Autodesk Inventor part; units mm, degrees
(part 2 of 3)
  line L643 (23.995, -22.9988) -> (23.995, -46.9725)
  line L644 (23.995, -46.9725) -> (32, -46.9725)
  line L645 (32, -46.9725) -> (40.005, -46.9725)
  line L646 (40.005, -46.9725) -> (41.9959, -46.9725)
  line L647 (41.9959, -46.9725) -> (48.01, -40.9997)
  line L648 (48.01, -40.9997) -> (48.01, -22.9988)
  line L649 (32, -47.4798) -> (32.0841, -48.285)
  line L650 (32.0841, -48.285) -> (32.3378, -49.0047)
  line L651 (32.3378, -49.0047) -> (32.6769, -49.7258)
  line L652 (32.6769, -49.7258) -> (33.1857, -50.3187)
  line L653 (33.1857, -50.3187) -> (33.7786, -50.826)
  line L654 (33.7786, -50.826) -> (34.4983, -51.1652)
  line L655 (34.4983, -51.1652) -> (35.218, -51.4189)
  line L656 (35.218, -51.4189) -> (36.0232, -51.5044)
  line L657 (36.0232, -51.5044) -> (36.7856, -51.4189)
  line L658 (36.7856, -51.4189) -> (37.548, -51.1652)
  line L659 (37.548, -51.1652) -> (38.225, -50.826)
  line L660 (38.225, -50.826) -> (38.8606, -50.3187)
  line L661 (38.8606, -50.3187) -> (39.3266, -49.7258)
  line L662 (39.3266, -49.7258) -> (39.7085, -49.0047)
  line L663 (39.7085, -49.0047) -> (39.9195, -48.285)
  line L664 (39.9195, -48.285) -> (40.005, -47.4798)
  line L665 (40.005, -22.4915) -> (39.9195, -21.729)
  line L666 (39.9195, -21.729) -> (39.7085, -20.9666)
  line L667 (39.7085, -20.9666) -> (39.3266, -20.2455)
  line L668 (39.3266, -20.2455) -> (38.8606, -19.6526)
  line L669 (38.8606, -19.6526) -> (38.225, -19.1453)
  line L670 (38.225, -19.1453) -> (37.548, -18.8061)
  line L671 (37.548, -18.8061) -> (36.7856, -18.5524)
  line L672 (36.7856, -18.5524) -> (36.0232, -18.5096)
  line L673 (36.0232, -18.5096) -> (35.218, -18.5524)
  line L674 (35.218, -18.5524) -> (34.4983, -18.8061)
  line L675 (34.4983, -18.8061) -> (33.7786, -19.1453)
  line L676 (33.7786, -19.1453) -> (33.1857, -19.6526)
  line L677 (33.1857, -19.6526) -> (32.6769, -20.2455)
  line L678 (32.6769, -20.2455) -> (32.3378, -20.9666)
  line L679 (32.3378, -20.9666) -> (32.0841, -21.729)
  line L680 (32.0841, -21.729) -> (32, -22.4915)
  line L681 (40.005, -47.4798) -> (40.005, -46.9725)
  line L682 (32, -47.4798) -> (32, -46.9725)
  line L683 (40.005, -22.4915) -> (40.005, -22.9988)
  line L684 (32, -22.4915) -> (32, -22.9988)
  line L685 (-48.9834, -46.9725) -> (-40.9784, -46.9725)
  line L686 (-40.9784, -46.9725) -> (-32.9734, -46.9725)
  line L687 (-32.9734, -46.9725) -> (-25.0111, -46.9725)
  line L688 (-25.0111, -46.9725) -> (-25.0111, -22.9988)
  line L689 (-25.0111, -22.9988) -> (-32.9734, -22.9988)
  line L690 (-32.9734, -22.9988) -> (-40.9784, -22.9988)
  line L691 (-40.9784, -22.9988) -> (-43.012, -22.9988)
  line L692 (-43.012, -22.9988) -> (-48.9834, -28.9716)
  line L693 (-48.9834, -28.9716) -> (-48.9834, -46.9725)
  line L694 (-32.9734, -22.4915) -> (-33.0575, -21.729)
  line L695 (-33.0575, -21.729) -> (-33.3126, -20.9666)
  line L696 (-33.3126, -20.9666) -> (-33.6503, -20.2455)
  line L697 (-33.6503, -20.2455) -> (-34.1591, -19.6526)
  line L698 (-34.1591, -19.6526) -> (-34.752, -19.1453)
  line L699 (-34.752, -19.1453) -> (-35.4717, -18.8061)
  line L700 (-35.4717, -18.8061) -> (-36.1927, -18.5524)
  line L701 (-36.1927, -18.5524) -> (-36.9965, -18.5096)
  line L702 (-36.9965, -18.5096) -> (-37.759, -18.5524)
  line L703 (-37.759, -18.5524) -> (-38.5214, -18.8061)
  line L704 (-38.5214, -18.8061) -> (-39.1998, -19.1453)
  line L705 (-39.1998, -19.1453) -> (-39.8354, -19.6526)
  line L706 (-39.8354, -19.6526) -> (-40.3, -20.2455)
  line L707 (-40.3, -20.2455) -> (-40.6819, -20.9666)
  line L708 (-40.6819, -20.9666) -> (-40.8943, -21.729)
  line L709 (-40.8943, -21.729) -> (-40.9784, -22.4915)
  line L710 (-40.9784, -47.4798) -> (-40.8943, -48.285)
  line L711 (-40.8943, -48.285) -> (-40.6819, -49.0047)
  line L712 (-40.6819, -49.0047) -> (-40.3, -49.7258)
  line L713 (-40.3, -49.7258) -> (-39.8354, -50.3187)
  line L714 (-39.8354, -50.3187) -> (-39.1998, -50.826)
  line L715 (-39.1998, -50.826) -> (-38.5214, -51.1652)
  line L716 (-38.5214, -51.1652) -> (-37.759, -51.4189)
  line L717 (-37.759, -51.4189) -> (-36.9965, -51.5044)
  line L718 (-36.9965, -51.5044) -> (-36.1927, -51.4189)
  line L719 (-36.1927, -51.4189) -> (-35.4717, -51.1652)
  line L720 (-35.4717, -51.1652) -> (-34.752, -50.826)
  line L721 (-34.752, -50.826) -> (-34.1591, -50.3187)
  line L722 (-34.1591, -50.3187) -> (-33.6503, -49.7258)
  line L723 (-33.6503, -49.7258) -> (-33.3126, -49.0047)
  line L724 (-33.3126, -49.0047) -> (-33.0575, -48.285)
  line L725 (-33.0575, -48.285) -> (-32.9734, -47.4798)
  line L726 (-40.9784, -22.4915) -> (-40.9784, -22.9988)
  line L727 (-32.9734, -22.4915) -> (-32.9734, -22.9988)
  line L728 (-40.9784, -47.4798) -> (-40.9784, -46.9725)
  line L729 (-32.9734, -47.4798) -> (-32.9734, -46.9725)
  line L730 (-22.9775, -13.469) -> (-22.9775, 13.5103)
  line L731 (-22.9775, 13.5103) -> (-4.9766, 13.5103)
  line L732 (-4.9766, 13.5103) -> (-4.9766, -13.469)
  line L733 (-4.9766, -13.469) -> (-22.9775, -13.469)
  line L734 (-22.0027, -6.4801) -> (-18.9957, -6.4801)
  line L735 (-20.4778, -4.998) -> (-20.4778, -8.005)
  line L736 (-20.4778, 8.005) -> (-20.4778, 4.9979)
  line L737 (-2.9857, -15.333) -> (3.1553, -15.333)
  line L738 (3.1553, -15.333) -> (3.1553, -17.4935)
  line L739 (3.1553, -17.4935) -> (-2.9857, -17.4935)
  line L740 (-2.9857, -17.4935) -> (-2.9857, -15.333)
  line L741 (-0.7411, -15.5453) -> (-0.7411, -17.2812)
  line L742 (0.7838, -16.3919) -> (-0.7411, -15.5453)
  line L743 (-0.7411, -17.2812) -> (0.7838, -16.3919)
  line L744 (0.7838, -15.5453) -> (0.7838, -16.3919)
  line L745 (0.7838, -16.3919) -> (0.7838, -17.2812)
  line L746 (-4.1714, 19.4403) -> (-4.1714, 19.1866)
  line L747 (-4.1714, 19.1866) -> (-4.1714, 16.2637)
  line L748 (-4.1714, 16.2637) -> (0.2751, 16.2637)
  line L749 (0.2751, 16.2637) -> (0.2751, 19.4403)
  line L750 (0.2751, 19.4403) -> (-3.7909, 19.4403)
  line L751 (-3.7909, 19.4403) -> (-3.875, 19.4403)
  line L752 (-3.875, 19.4403) -> (-4.1714, 19.4403)
  line L753 (-3.875, 19.4403) -> (-3.875, 19.1866)
  line L754 (-3.875, 19.1866) -> (-4.1714, 19.1866)
  line L755 (-3.7909, 19.4403) -> (-3.7909, 19.1439)
  line L756 (-3.7909, 19.1439) -> (-4.0873, 19.1439)
  line L757 (64.104, 31.9772) -> (64.104, 33.6717)
  line L758 (50.6351, 31.9772) -> (50.6351, 33.6717)
  line L759 (64.104, 14.1032) -> (63.1307, 14.1032)
  line L760 (64.104, 14.1032) -> (64.104, 15.0779)
  line L761 (50.6351, 14.1032) -> (51.6099, 14.1032)
  line L762 (50.6351, 14.1032) -> (50.6351, 15.0779)
  line L763 (50.6351, 39.8981) -> (51.6099, 39.8981)
  line L764 (50.6351, 39.8981) -> (50.6351, 38.882)
  line L765 (64.104, 39.8981) -> (63.0038, 39.8981)
  line L766 (64.104, 39.8981) -> (64.104, 38.882)
  line L767 (-5.9927, -49.9795) -> (5.9941, -49.9795)
  line L768 (5.9941, -49.9795) -> (5.9941, -48.9634)
  line L769 (5.9941, -48.9634) -> (5.9941, -38.9675)
  line L770 (5.9941, -38.9675) -> (5.9941, -29.9877)
  line L771 (5.9941, -29.9877) -> (-5.9927, -29.9877)
  line L772 (-5.9927, -29.9877) -> (-5.9927, -38.9675)
  line L773 (-5.9927, -38.9675) -> (-5.9927, -48.9634)
  line L774 (-5.9927, -48.9634) -> (-5.9927, -49.9795)
  line L775 (-8.9998, -38.9675) -> (-9.8477, -39.0516)
  line L776 (-9.8477, -39.0516) -> (-10.6942, -39.2639)
  line L777 (-10.6942, -39.2639) -> (-11.4994, -39.6444)
  line L778 (-11.4994, -39.6444) -> (-12.2191, -40.1532)
  line L779 (-12.2191, -40.1532) -> (-12.812, -40.746)
  line L780 (-12.812, -40.746) -> (-13.3207, -41.4658)
  line L781 (-13.3207, -41.4658) -> (-13.7013, -42.2709)
  line L782 (-13.7013, -42.2709) -> (-13.9136, -43.1175)
  line L783 (-13.9136, -43.1175) -> (-13.9977, -43.9654)
  line L784 (-13.9977, -43.9654) -> (-13.9136, -44.8547)
  line L785 (-13.9136, -44.8547) -> (-13.7013, -45.7013)
  line L786 (-13.7013, -45.7013) -> (-13.3207, -46.4637)
  line L787 (-13.3207, -46.4637) -> (-12.812, -47.1834)
  line L788 (-12.812, -47.1834) -> (-12.2191, -47.819)
  line L789 (-12.2191, -47.819) -> (-11.4994, -48.3278)
  line L790 (-11.4994, -48.3278) -> (-10.6942, -48.6669)
  line L791 (-10.6942, -48.6669) -> (-9.8477, -48.9206)
  line L792 (-9.8477, -48.9206) -> (-8.9998, -48.9634)
  line L793 (9.0011, -48.9634) -> (9.8904, -48.9206)
  line L794 (9.8904, -48.9206) -> (10.737, -48.6669)
  line L795 (10.737, -48.6669) -> (11.4994, -48.3278)
  line L796 (11.4994, -48.3278) -> (12.2191, -47.819)
  line L797 (12.2191, -47.819) -> (12.8547, -47.1834)
  line L798 (12.8547, -47.1834) -> (13.3635, -46.4637)
  line L799 (13.3635, -46.4637) -> (13.7027, -45.7013)
  line L800 (13.7027, -45.7013) -> (13.9563, -44.8547)
  line L801 (13.9563, -44.8547) -> (13.9991, -43.9654)
  line L802 (13.9991, -43.9654) -> (13.9563, -43.1175)
  line L803 (13.9563, -43.1175) -> (13.7027, -42.2709)
  line L804 (13.7027, -42.2709) -> (13.3635, -41.4658)
  line L805 (13.3635, -41.4658) -> (12.8547, -40.746)
  line L806 (12.8547, -40.746) -> (12.2191, -40.1532)
  line L807 (12.2191, -40.1532) -> (11.4994, -39.6444)
  line L808 (11.4994, -39.6444) -> (10.737, -39.2639)
  line L809 (10.737, -39.2639) -> (9.8904, -39.0516)
  line L810 (9.8904, -39.0516) -> (9.0011, -38.9675)
  line L811 (-8.9998, -38.9675) -> (-5.9927, -38.9675)
  line L812 (-8.9998, -48.9634) -> (-5.9927, -48.9634)
  line L813 (5.9941, -38.9675) -> (9.0011, -38.9675)
  line L814 (5.9941, -48.9634) -> (9.0011, -48.9634)
  line L815 (-7.4749, -49.9795) -> (-7.4749, -38.4587)
  line L816 (-7.4749, -38.4587) -> (7.5176, -38.4587)
  line L817 (7.5176, -38.4587) -> (7.5176, -49.9795)
  line L818 (7.5176, -49.9795) -> (-7.4749, -49.9795)
  line L819 (5.9941, 49.9781) -> (-5.9927, 49.9781)
  line L820 (-5.9927, 49.9781) -> (-5.9927, 49.0047)
  line L821 (-5.9927, 49.0047) -> (-5.9927, 39.0088)
  line L822 (-5.9927, 39.0088) -> (-5.9927, 29.9863)
  line L823 (-5.9927, 29.9863) -> (5.9941, 29.9863)
  line L824 (5.9941, 29.9863) -> (5.9941, 39.0088)
  line L825 (5.9941, 39.0088) -> (5.9941, 49.0047)
  line L826 (5.9941, 49.0047) -> (5.9941, 49.9781)
  line L827 (9.0011, 39.0088) -> (9.8904, 39.0929)
  line L828 (9.8904, 39.0929) -> (10.737, 39.3053)
  line L829 (10.737, 39.3053) -> (11.4994, 39.6858)
  line L830 (11.4994, 39.6858) -> (12.2191, 40.1518)
  line L831 (12.2191, 40.1518) -> (12.8547, 40.7874)
  line L832 (12.8547, 40.7874) -> (13.3635, 41.5071)
  line L833 (13.3635, 41.5071) -> (13.7027, 42.2696)
  line L834 (13.7027, 42.2696) -> (13.9563, 43.1175)
  line L835 (13.9563, 43.1175) -> (13.9991, 44.0068)
  line L836 (13.9991, 44.0068) -> (13.9563, 44.8533)
  line L837 (13.9563, 44.8533) -> (13.7027, 45.7013)
  line L838 (13.7027, 45.7013) -> (13.3635, 46.5051)
  line L839 (13.3635, 46.5051) -> (12.8547, 47.2261)
  line L840 (12.8547, 47.2261) -> (12.2191, 47.819)
  line L841 (12.2191, 47.819) -> (11.4994, 48.3264)
  line L842 (11.4994, 48.3264) -> (10.737, 48.7083)
  line L843 (10.737, 48.7083) -> (9.8904, 48.9192)
  line L844 (9.8904, 48.9192) -> (9.0011, 49.0047)
  line L845 (-8.9998, 49.0047) -> (-9.8477, 48.9192)
  line L846 (-9.8477, 48.9192) -> (-10.6942, 48.7083)
  line L847 (-10.6942, 48.7083) -> (-11.4994, 48.3264)
  line L848 (-11.4994, 48.3264) -> (-12.2191, 47.819)
  line L849 (-12.2191, 47.819) -> (-12.812, 47.2261)
  line L850 (-12.812, 47.2261) -> (-13.3207, 46.5051)
  line L851 (-13.3207, 46.5051) -> (-13.7013, 45.7013)
  line L852 (-13.7013, 45.7013) -> (-13.9136, 44.8533)
  line L853 (-13.9136, 44.8533) -> (-13.9977, 44.0068)
  line L854 (-13.9977, 44.0068) -> (-13.9136, 43.1175)
  line L855 (-13.9136, 43.1175) -> (-13.7013, 42.2696)
  line L856 (-13.7013, 42.2696) -> (-13.3207, 41.5071)
  line L857 (-13.3207, 41.5071) -> (-12.812, 40.7874)
  line L858 (-12.812, 40.7874) -> (-12.2191, 40.1518)
  line L859 (-12.2191, 40.1518) -> (-11.4994, 39.6858)
  line L860 (-11.4994, 39.6858) -> (-10.6942, 39.3053)
  line L861 (-10.6942, 39.3053) -> (-9.8477, 39.0929)
  line L862 (-9.8477, 39.0929) -> (-8.9998, 39.0088)
  line L863 (9.0011, 39.0088) -> (5.9941, 39.0088)
  line L864 (9.0011, 49.0047) -> (5.9941, 49.0047)
  line L865 (-5.9927, 39.0088) -> (-8.9998, 39.0088)
  line L866 (-5.9927, 49.0047) -> (-8.9998, 49.0047)
  line L867 (7.5176, 49.9781) -> (7.5176, 38.5001)
  line L868 (7.5176, 38.5001) -> (-7.4749, 38.5001)
  line L869 (-7.4749, 38.5001) -> (-7.4749, 49.9781)
  line L870 (-7.4749, 49.9781) -> (7.5176, 49.9781)
  line L871 (29.2894, -9.1066) -> (32.5928, -9.1066)
  line L872 (32.5928, -9.1066) -> (32.5928, -14.3169)
  line L873 (32.5928, -14.3169) -> (29.2894, -14.3169)
  line L874 (29.2894, -14.3169) -> (29.2894, -9.1066)
  line L875 (31.0679, -4.1941) -> (31.0679, 2.7947)
  line L876 (31.0679, 2.7947) -> (38.0568, 2.7947)
  line L877 (38.0568, 2.7947) -> (38.0568, -3.855)
  line L878 (37.7176, -4.1941) -> (31.0679, -4.1941)
  line L879 (37.7176, -4.1941) -> (38.0568, -3.855)
  line L880 (58.0472, -22.5328) -> (68.2554, -22.5328)
  line L881 (68.2554, -22.5328) -> (68.2554, -17.3239)
  line L882 (68.2554, -17.3239) -> (58.0472, -17.3239)
  line L883 (58.0472, -17.3653) -> (58.0472, -21.1775)
  line L884 (58.0472, -21.1775) -> (58.0472, -22.4487)
  line L885 (59.3184, -22.4487) -> (59.3184, -21.1775)
  line L886 (59.3184, -21.1775) -> (58.0472, -21.1775)
  line L887 (68.0018, -3.9818) -> (68.0018, -1.1016)
  line L888 (68.0018, -1.1016) -> (69.8644, -1.1016)
  line L889 (69.8644, -1.1016) -> (69.8644, -3.9818)
  line L890 (69.8644, -3.9818) -> (68.0018, -3.9818)
  line L891 (49.2798, 0.1696) -> (49.1957, 0.6356)
  line L892 (49.1957, 0.6356) -> (49.0261, 1.1002)
  line L893 (49.0261, 1.1002) -> (48.7724, 1.5249)
  line L894 (48.7724, 1.5249) -> (48.3905, 1.8213)
  line L895 (48.3905, 2.4555) -> (49.408, 2.4555)
  line L896 (48.3905, -8.3869) -> (48.7724, -8.0477)
  line L897 (48.7724, -8.0477) -> (49.0261, -7.6672)
  line L898 (49.0261, -7.6672) -> (49.1957, -7.2012)
  line L899 (49.1957, -7.2012) -> (49.2798, -6.6924)
  line L900 (48.3905, -8.9798) -> (49.408, -8.9798)
  line L901 (45.9763, -6.6924) -> (45.9763, 0.1696)
  line L902 (45.2139, -6.6924) -> (45.2139, 0.1696)
  line L903 (48.5173, 0.1696) -> (48.5173, -6.6924)
  line L904 (44.8333, -8.7261) -> (44.8333, 2.2019)
  line L905 (44.8333, -8.7261) -> (44.8747, -8.8529)
  line L906 (44.8747, -8.8529) -> (44.9602, -8.937)
  line L907 (44.9602, -8.937) -> (45.087, -8.9798)
  line L908 (45.087, -8.9798) -> (46.1032, -8.9798)
  line L909 (45.9763, -6.6924) -> (46.0191, -6.9889)
  line L910 (46.0191, -6.9889) -> (46.1032, -7.2425)
  line L911 (48.3905, -7.2425) -> (48.476, -6.9889)
  line L912 (48.476, -6.9889) -> (48.5173, -6.6924)
  line L913 (45.2139, -6.6924) -> (45.2566, -7.2012)
  line L914 (45.2566, -7.2012) -> (45.4262, -7.6672)
  line L915 (45.4262, -7.6672) -> (45.7226, -8.0477)
  line L916 (45.7226, -8.0477) -> (46.1032, -8.3869)
  line L917 (46.1032, 1.8213) -> (45.7226, 1.5249)
  line L918 (45.7226, 1.5249) -> (45.4262, 1.1002)
  line L919 (45.4262, 1.1002) -> (45.2566, 0.6356)
  line L920 (45.2566, 0.6356) -> (45.2139, 0.1696)
  line L921 (46.1032, 0.7197) -> (46.0191, 0.466)
  line L922 (46.0191, 0.466) -> (45.9763, 0.1696)
  line L923 (48.5173, 0.1696) -> (48.476, 0.466)
  line L924 (48.476, 0.466) -> (48.3905, 0.7197)
  line L925 (45.087, 2.4555) -> (46.1032, 2.4555)
  line L926 (45.087, 2.4555) -> (44.9602, 2.4142)
  line L927 (44.9602, 2.4142) -> (44.8747, 2.3287)
  line L928 (44.8747, 2.3287) -> (44.8333, 2.2019)
  line L929 (49.2798, 0.1696) -> (49.2798, -6.6924)
  line L930 (49.6617, -8.7261) -> (49.6617, 2.2019)
  line L931 (49.408, -8.9798) -> (49.5349, -8.937)
  line L932 (49.5349, -8.937) -> (49.619, -8.8529)
  line L933 (49.619, -8.8529) -> (49.6617, -8.7261)
  line L934 (49.6617, 2.2019) -> (49.619, 2.3287)
  line L935 (49.619, 2.3287) -> (49.5349, 2.4142)
  line L936 (49.5349, 2.4142) -> (49.408, 2.4555)
  line L937 (46.6119, -3.5158) -> (47.8831, -3.5158)
  line L938 (47.8831, -3.5158) -> (47.8831, -3.007)
  line L939 (47.8831, -3.007) -> (46.6119, -3.007)
  line L940 (46.6119, -3.007) -> (46.6119, -3.5158)
  line L941 (46.6119, -3.8977) -> (47.2475, -3.8977)
  line L942 (47.2475, -3.8977) -> (47.8831, -3.8977)
  line L943 (47.2475, -3.8977) -> (47.2475, -4.4051)
  line L944 (46.6119, -2.6265) -> (47.2475, -2.6265)
  line L945 (47.2475, -2.6265) -> (47.8831, -2.6265)
  line L946 (47.2475, -2.6265) -> (47.2475, -2.1178)
  line L947 (56.7347, -5.5908) -> (56.7347, -11.6904)
  line L948 (56.7347, -11.6904) -> (54.5328, -11.6904)
  line L949 (54.5328, -11.6904) -> (54.5328, -5.5908)
  line L950 (54.5328, -5.5908) -> (56.7347, -5.5908)
  line L951 (56.5223, -7.8354) -> (54.7437, -7.8354)
  line L952 (55.633, -9.3603) -> (56.5223, -7.8354)
  line L953 (54.7437, -7.8354) -> (55.633, -9.3603)
  line L954 (56.5223, -9.3603) -> (55.633, -9.3603)
  line L955 (55.633, -9.3603) -> (54.7437, -9.3603)
  line L956 (61.1825, -5.6763) -> (61.1825, -11.7745)
  line L957 (61.1825, -11.7745) -> (58.9793, -11.7745)
  line L958 (58.9793, -11.7745) -> (58.9793, -5.6763)
  line L959 (58.9793, -5.6763) -> (61.1825, -5.6763)
  line L960 (60.9702, -7.8781) -> (59.1916, -7.8781)
  line L961 (60.0809, -9.403) -> (60.9702, -7.8781)
  line L962 (59.1916, -7.8781) -> (60.0809, -9.403)
  line L963 (60.9702, -9.403) -> (60.0809, -9.403)
  line L964 (60.0809, -9.403) -> (59.1916, -9.403)
  line L965 (-17.3867, -28.2932) -> (-13.7013, -28.2932)
  line L966 (-13.7013, -28.2932) -> (-13.7013, -21.6008)
  line L967 (-13.7013, -21.6008) -> (-17.3867, -21.6008)
  line L968 (-17.3867, -21.6008) -> (-17.3867, -28.2932)
  line L969 (-42.4178, -1.4822) -> (-42.4178, 4.616)
  line L970 (-42.4178, 4.616) -> (-40.2159, 4.616)
  line L971 (-40.2159, 4.616) -> (-40.2159, -1.4822)
  line L972 (-40.2159, -1.4822) -> (-42.4178, -1.4822)
  line L973 (-42.2068, 0.7624) -> (-40.4282, 0.7624)
  line L974 (-41.3175, 2.2873) -> (-42.2068, 0.7624)
  line L975 (-40.4282, 0.7624) -> (-41.3175, 2.2873)
  spline S88 degree 3 poles (-31.4912, -11.9868) (-31.4912, -12.792) (-32.1682, -13.469) (-32.9734, -13.469) knots 0 0 0 0 1 1 1 1
  line L976 (-31.4912, -11.9868) -> (-31.4912, -12.792) construction
  line L977 (-31.4912, -12.792) -> (-32.1682, -13.469) construction
  line L978 (-32.1682, -13.469) -> (-32.9734, -13.469) construction
  spline S89 degree 3 poles (-32.9734, -13.469) (-33.7786, -13.469) (-34.4555, -12.792) (-34.4555, -11.9868) knots 0 0 0 0 1 1 1 1
  line L979 (-32.9734, -13.469) -> (-33.7786, -13.469) construction
  line L980 (-33.7786, -13.469) -> (-34.4555, -12.792) construction
  line L981 (-34.4555, -12.792) -> (-34.4555, -11.9868) construction
  spline S90 degree 3 poles (-34.4555, -11.9868) (-34.4555, -11.1816) (-33.7786, -10.5047) (-32.9734, -10.5047) knots 0 0 0 0 1 1 1 1
  line L982 (-34.4555, -11.9868) -> (-34.4555, -11.1816) construction
  line L983 (-34.4555, -11.1816) -> (-33.7786, -10.5047) construction
  line L984 (-33.7786, -10.5047) -> (-32.9734, -10.5047) construction
  spline S91 degree 3 poles (-32.9734, -10.5047) (-32.1682, -10.5047) (-31.4912, -11.1816) (-31.4912, -11.9868) knots 0 0 0 0 1 1 1 1
  line L985 (-32.9734, -10.5047) -> (-32.1682, -10.5047) construction
  line L986 (-32.1682, -10.5047) -> (-31.4912, -11.1816) construction
  line L987 (-31.4912, -11.1816) -> (-31.4912, -11.9868) construction
  line L988 (-42.2068, 2.2873) -> (-41.3175, 2.2873)
  line L989 (-41.3175, 2.2873) -> (-40.4282, 2.2873)
  spline S92 degree 3 poles (-31.4912, 12.0282) (-31.4912, 11.2244) (-32.1682, 10.546) (-32.9734, 10.546) knots 0 0 0 0 1 1 1 1
  line L990 (-31.4912, 12.0282) -> (-31.4912, 11.2244) construction
  line L991 (-31.4912, 11.2244) -> (-32.1682, 10.546) construction
  line L992 (-32.1682, 10.546) -> (-32.9734, 10.546) construction
  spline S93 degree 3 poles (-32.9734, 10.546) (-33.7786, 10.546) (-34.4555, 11.2244) (-34.4555, 12.0282) knots 0 0 0 0 1 1 1 1
  line L993 (-32.9734, 10.546) -> (-33.7786, 10.546) construction
  line L994 (-33.7786, 10.546) -> (-34.4555, 11.2244) construction
  line L995 (-34.4555, 11.2244) -> (-34.4555, 12.0282) construction
  spline S94 degree 3 poles (-34.4555, 12.0282) (-34.4555, 12.8334) (-33.7786, 13.5103) (-32.9734, 13.5103) knots 0 0 0 0 1 1 1 1
  line L996 (-34.4555, 12.0282) -> (-34.4555, 12.8334) construction
  line L997 (-34.4555, 12.8334) -> (-33.7786, 13.5103) construction
  line L998 (-33.7786, 13.5103) -> (-32.9734, 13.5103) construction
  spline S95 degree 3 poles (-32.9734, 13.5103) (-32.1682, 13.5103) (-31.4912, 12.8334) (-31.4912, 12.0282) knots 0 0 0 0 1 1 1 1
  line L999 (-32.9734, 13.5103) -> (-32.1682, 13.5103) construction
  line L1000 (-32.1682, 13.5103) -> (-31.4912, 12.8334) construction
  line L1001 (-31.4912, 12.8334) -> (-31.4912, 12.0282) construction
  line L1002 (-30.0077, -16.9848) -> (-30.0077, -6.9889)
  line L1003 (-30.0077, -6.9889) -> (-35.9804, -6.9889)
  line L1004 (-35.9804, -6.9889) -> (-35.9804, -16.9848)
  line L1005 (-35.9804, -16.9848) -> (-30.0077, -16.9848)
  spline S96 degree 3 poles (-31.4912, 0) (-31.4912, -0.8052) (-32.1682, -1.4822) (-32.9734, -1.4822) knots 0 0 0 0 1 1 1 1
  line L1006 (-31.4912, 0) -> (-31.4912, -0.8052) construction
  line L1007 (-31.4912, -0.8052) -> (-32.1682, -1.4822) construction
  line L1008 (-32.1682, -1.4822) -> (-32.9734, -1.4822) construction
  spline S97 degree 3 poles (-32.9734, -1.4822) (-33.7786, -1.4822) (-34.4555, -0.8052) (-34.4555, 0) knots 0 0 0 0 1 1 1 1
  line L1009 (-32.9734, -1.4822) -> (-33.7786, -1.4822) construction
  line L1010 (-33.7786, -1.4822) -> (-34.4555, -0.8052) construction
  line L1011 (-34.4555, -0.8052) -> (-34.4555, 0) construction
  spline S98 degree 3 poles (-34.4555, 0) (-34.4555, 0.8038) (-33.7786, 1.4821) (-32.9734, 1.4821) knots 0 0 0 0 1 1 1 1
  line L1012 (-34.4555, 0) -> (-34.4555, 0.8038) construction
  line L1013 (-34.4555, 0.8038) -> (-33.7786, 1.4821) construction
  line L1014 (-33.7786, 1.4821) -> (-32.9734, 1.4821) construction
  spline S99 degree 3 poles (-32.9734, 1.4821) (-32.1682, 1.4821) (-31.4912, 0.8038) (-31.4912, 0) knots 0 0 0 0 1 1 1 1
  line L1015 (-32.9734, 1.4821) -> (-32.1682, 1.4821) construction
  line L1016 (-32.1682, 1.4821) -> (-31.4912, 0.8038) construction
  line L1017 (-31.4912, 0.8038) -> (-31.4912, 0) construction
  line L1018 (-30.0077, 7.0302) -> (-30.0077, 17.0261)
  line L1019 (-30.0077, 17.0261) -> (-35.9804, 17.0261)
  line L1020 (-35.9804, 17.0261) -> (-35.9804, 7.0302)
  line L1021 (-35.9804, 7.0302) -> (-30.0077, 7.0302)
  line L1022 (-30.0077, -4.998) -> (-30.0077, 4.9979)
  line L1023 (-30.0077, 4.9979) -> (-35.9804, 4.9979)
  line L1024 (-35.9804, 4.9979) -> (-35.9804, -4.998)
  line L1025 (-35.9804, -4.998) -> (-30.0077, -4.998)
  line L1026 (66.2645, 19.3976) -> (72.3641, 19.3976)
  line L1027 (72.3641, 19.3976) -> (72.3641, 17.1957)
  line L1028 (72.3641, 17.1957) -> (66.2645, 17.1957)
  line L1029 (66.2645, 17.1957) -> (66.2645, 19.3976)
  line L1030 (68.5091, 19.1866) -> (68.5091, 17.408)
  line L1031 (70.034, 18.2973) -> (68.5091, 19.1866)
  line L1032 (68.5091, 17.408) -> (70.034, 18.2973)
  line L1033 (70.034, 19.1866) -> (70.034, 18.2973)
  line L1034 (70.034, 18.2973) -> (70.034, 17.408)
  line L1035 (66.561, 12.6638) -> (72.6605, 12.6638)
  line L1036 (72.6605, 12.6638) -> (72.6605, 10.4619)
  line L1037 (72.6605, 10.4619) -> (66.561, 10.4619)
  line L1038 (66.561, 10.4619) -> (66.561, 12.6638)
  line L1039 (68.8056, 12.4514) -> (68.8056, 10.6729)
  line L1040 (70.3305, 11.5621) -> (68.8056, 12.4514)
  line L1041 (68.8056, 10.6729) -> (70.3305, 11.5621)
  line L1042 (70.3305, 12.4514) -> (70.3305, 11.5621)
  line L1043 (70.3305, 11.5621) -> (70.3305, 10.6729)
  line L1044 (51.7794, -27.9968) -> (51.7794, -44.5155)
  line L1045 (58.1754, -44.5155) -> (51.7794, -44.5155)
  line L1046 (58.1754, -44.5155) -> (58.1754, -27.9968)
  line L1047 (51.7794, -27.9968) -> (58.1754, -27.9968)
  line L1048 (57.0311, -29.1412) -> (57.0311, -30.666)
  line L1049 (52.9652, -30.666) -> (52.9652, -29.1412)
  line L1050 (57.0311, -30.666) -> (52.9652, -30.666)
  line L1051 (52.9652, -29.1412) -> (57.0311, -29.1412)
  line L1052 (57.0311, -31.6822) -> (57.0311, -33.2071)
  line L1053 (52.9652, -33.2071) -> (52.9652, -31.6822)
  line L1054 (57.0311, -33.2071) -> (52.9652, -33.2071)
  line L1055 (52.9652, -31.6822) -> (57.0311, -31.6822)
  line L1056 (57.0311, -34.2232) -> (57.0311, -35.7481)
  line L1057 (52.9652, -35.7481) -> (52.9652, -34.2232)
  line L1058 (57.0311, -35.7481) -> (52.9652, -35.7481)
  line L1059 (52.9652, -34.2232) -> (57.0311, -34.2232)
  line L1060 (57.0311, -36.7642) -> (57.0311, -38.2891)
  line L1061 (52.9652, -38.2891) -> (52.9652, -36.7642)
  line L1062 (57.0311, -38.2891) -> (52.9652, -38.2891)
  line L1063 (52.9652, -36.7642) -> (57.0311, -36.7642)
  line L1064 (57.0311, -39.3053) -> (57.0311, -40.8301)
  line L1065 (52.9652, -40.8301) -> (52.9652, -39.3053)
  line L1066 (57.0311, -40.8301) -> (52.9652, -40.8301)
  line L1067 (52.9652, -39.3053) -> (57.0311, -39.3053)
  line L1068 (57.0311, -41.8477) -> (57.0311, -43.3726)
  line L1069 (52.9652, -43.3726) -> (52.9652, -41.8477)
  line L1070 (57.0311, -43.3726) -> (52.9652, -43.3726)
  line L1071 (52.9652, -41.8477) -> (57.0311, -41.8477)
  line L1072 (-10.8211, 30.2841) -> (-10.8211, 34.0109)
  line L1073 (-10.8211, 34.0109) -> (-17.5135, 34.0109)
  line L1074 (-17.5135, 34.0109) -> (-17.5135, 30.2841)
  line L1075 (-17.5135, 30.2841) -> (-10.8211, 30.2841)
  line L1076 (14.2955, -22.7879) -> (12.0082, -22.7879)
  line L1077 (12.0082, -31.5553) -> (12.8547, -31.5553)
  line L1078 (12.8547, -31.5553) -> (13.4476, -31.5553)
  line L1079 (13.4476, -31.5553) -> (14.2955, -31.5553)
  line L1080 (37.6321, 59.5935) -> (38.6497, 59.5935)
  line L1081 (35.9391, 62.7701) -> (33.9895, 62.7701)
  line L1082 (33.3966, 62.7701) -> (31.4485, 62.7701)
  line L1083 (33.3966, 62.7701) -> (33.4394, 62.5578)
  line L1084 (33.4394, 62.5578) -> (33.609, 62.4737)
  line L1085 (33.609, 62.4737) -> (33.7786, 62.4737)
  line L1086 (33.7786, 62.4737) -> (33.9481, 62.5578)
  line L1087 (33.9481, 62.5578) -> (33.9895, 62.7701)
  line L1088 (33.3966, 62.7701) -> (33.4394, 62.5578)
  line L1089 (33.4394, 62.5578) -> (33.609, 62.4737)
  line L1090 (33.609, 62.4737) -> (33.7786, 62.4737)
  line L1091 (33.7786, 62.4737) -> (33.9481, 62.5578)
  line L1092 (33.9481, 62.5578) -> (33.9895, 62.7701)
  line L1093 (37.7176, 59.5507) -> (38.7338, 59.5507)
  line L1094 (31.4485, 57.6867) -> (35.9391, 57.6867)
  line L1095 (33.9895, 62.7701) -> (33.3966, 62.7701)
  line L1096 (33.3966, 62.7701) -> (33.4394, 62.5578)
  line L1097 (33.4394, 62.5578) -> (33.609, 62.4737)
  line L1098 (33.609, 62.4737) -> (33.7786, 62.4737)
  line L1099 (33.7786, 62.4737) -> (33.9481, 62.5578)
  line L1100 (33.9481, 62.5578) -> (33.9895, 62.7701)
  line L1101 (67.6198, 2.1178) -> (67.6198, 0.5074)
  line L1102 (65.2057, 2.1178) -> (65.2057, 0.5074)
  line L1103 (68.0018, 1.9909) -> (67.9163, 1.9909)
  line L1104 (67.9163, 1.9909) -> (67.9163, 2.1178)
  line L1105 (3.8763, 32.2737) -> (5.1462, 32.2737)
  line L1106 (5.1462, 32.2737) -> (5.7818, 31.6394)
  line L1107 (5.7818, 31.6394) -> (5.7818, 30.3682)
  line L1108 (5.7818, 30.3682) -> (5.1462, 29.7326)
  line L1109 (3.2407, 31.6394) -> (3.2407, 30.3682)
  line L1110 (3.8763, 32.2737) -> (3.2407, 31.6394)
  line L1111 (3.2407, 30.3682) -> (3.8763, 29.7326)
  line L1112 (5.1462, 29.7326) -> (3.8763, 29.7326)
  line L1113 (-5.1034, 32.2737) -> (-3.8336, 32.2737)
  line L1114 (-3.8336, 32.2737) -> (-3.2394, 31.6394)
  line L1115 (-3.2394, 31.6394) -> (-3.2394, 30.3682)
  line L1116 (-3.2394, 30.3682) -> (-3.8336, 29.7326)
  line L1117 (-5.739, 31.6394) -> (-5.739, 30.3682)
  line L1118 (-5.1034, 32.2737) -> (-5.739, 31.6394)
  line L1119 (-5.739, 30.3682) -> (-5.1034, 29.7326)
  line L1120 (-3.8336, 29.7326) -> (-5.1034, 29.7326)
  line L1121 (-5.1034, -29.734) -> (-3.8336, -29.734)
  line L1122 (-3.8336, -29.734) -> (-3.2394, -30.3696)
  line L1123 (-3.2394, -30.3696) -> (-3.2394, -31.6394)
  line L1124 (-3.2394, -31.6394) -> (-3.8336, -32.275)
  line L1125 (-5.739, -30.3696) -> (-5.739, -31.6394)
  line L1126 (-5.1034, -29.734) -> (-5.739, -30.3696)
  line L1127 (-5.739, -31.6394) -> (-5.1034, -32.275)
  line L1128 (-3.8336, -32.275) -> (-5.1034, -32.275)
  line L1129 (3.8763, -29.734) -> (5.1462, -29.734)
  line L1130 (5.1462, -29.734) -> (5.7818, -30.3696)
  line L1131 (5.7818, -30.3696) -> (5.7818, -31.6394)
  line L1132 (5.7818, -31.6394) -> (5.1462, -32.275)
  line L1133 (3.2407, -30.3696) -> (3.2407, -31.6394)
  line L1134 (3.8763, -29.734) -> (3.2407, -30.3696)
  line L1135 (3.2407, -31.6394) -> (3.8763, -32.275)
  line L1136 (5.1462, -32.275) -> (3.8763, -32.275)
  line L1137 (3.0712, 17.7045) -> (3.664, 17.7045)
  line L1138 (3.664, 17.7045) -> (4.341, 17.7045)
  line L1139 (4.341, 17.7045) -> (4.9766, 17.7045)
  line L1140 (4.9766, 17.7045) -> (4.9766, 14.3155)
  line L1141 (4.9766, 14.3155) -> (4.341, 14.3155)
  line L1142 (4.341, 14.3155) -> (3.664, 14.3155)
  line L1143 (3.664, 14.3155) -> (3.0712, 14.3155)
  line L1144 (3.0712, 14.3155) -> (3.0712, 17.7045)
  line L1145 (4.7656, 16.3064) -> (3.3248, 16.3064)
  line L1146 (3.664, 17.7045) -> (3.7068, 17.5349)
  line L1147 (3.7068, 17.5349) -> (3.8336, 17.408)
  line L1148 (3.8336, 17.408) -> (4.0032, 17.3653)
  line L1149 (4.0032, 17.3653) -> (4.1728, 17.408)
  line L1150 (4.1728, 17.408) -> (4.2996, 17.5349)
  line L1151 (4.2996, 17.5349) -> (4.341, 17.7045)
  line L1152 (4.341, 14.3155) -> (4.2996, 14.4851)
  line L1153 (4.2996, 14.4851) -> (4.1728, 14.6119)
  line L1154 (4.1728, 14.6119) -> (4.0032, 14.6547)
  line L1155 (4.0032, 14.6547) -> (3.8336, 14.6119)
  line L1156 (3.8336, 14.6119) -> (3.7068, 14.4851)
  line L1157 (3.7068, 14.4851) -> (3.664, 14.3155)
  line L1158 (-30.686, -50.9529) -> (-30.686, -50.3187)
  line L1159 (-30.686, -50.3187) -> (-30.686, -49.6403)
  line L1160 (-30.686, -49.6403) -> (-30.686, -49.0475)
  line L1161 (-30.686, -49.0475) -> (-27.2971, -49.0475)
  line L1162 (-27.2971, -49.0475) -> (-27.2971, -49.6403)
  line L1163 (-27.2971, -49.6403) -> (-27.2971, -50.3187)
  line L1164 (-27.2971, -50.3187) -> (-27.2971, -50.9529)
  line L1165 (-27.2971, -50.9529) -> (-30.686, -50.9529)
  line L1166 (-29.288, -49.2171) -> (-29.288, -50.6992)
  line L1167 (-30.686, -50.3187) -> (-30.5164, -50.2759)
  line L1168 (-30.5164, -50.2759) -> (-30.3896, -50.1491)
  line L1169 (-30.3896, -50.1491) -> (-30.3469, -49.9795)
  line L1170 (-30.3469, -49.9795) -> (-30.3896, -49.8099)
  line L1171 (-30.3896, -49.8099) -> (-30.5164, -49.6831)
  line L1172 (-30.5164, -49.6831) -> (-30.686, -49.6403)
  line L1173 (-27.2971, -49.6403) -> (-27.4667, -49.6831)
  line L1174 (-27.4667, -49.6831) -> (-27.5935, -49.8099)
  line L1175 (-27.5935, -49.8099) -> (-27.6363, -49.9795)
  line L1176 (-27.6363, -49.9795) -> (-27.5935, -50.1491)
  line L1177 (-27.5935, -50.1491) -> (-27.4667, -50.2759)
  line L1178 (-27.4667, -50.2759) -> (-27.2971, -50.3187)
  line L1179 (-30.686, -53.9186) -> (-30.686, -53.3257)
  line L1180 (-30.686, -53.3257) -> (-30.686, -52.6474)
  line L1181 (-30.686, -52.6474) -> (-30.686, -52.0545)
  line L1182 (-30.686, -52.0545) -> (-27.2971, -52.0545)
  line L1183 (-27.2971, -52.0545) -> (-27.2971, -52.6474)
  line L1184 (-27.2971, -52.6474) -> (-27.2971, -53.3257)
  line L1185 (-27.2971, -53.3257) -> (-27.2971, -53.9186)
  line L1186 (-27.2971, -53.9186) -> (-30.686, -53.9186)
  line L1187 (-29.288, -52.2241) -> (-29.288, -53.7062)
  line L1188 (-30.686, -53.3257) -> (-30.5164, -53.283)
  line L1189 (-30.5164, -53.283) -> (-30.3896, -53.1561)
  line L1190 (-30.3896, -53.1561) -> (-30.3469, -52.9865)
  line L1191 (-30.3469, -52.9865) -> (-30.3896, -52.817)
  line L1192 (-30.3896, -52.817) -> (-30.5164, -52.6901)
  line L1193 (-30.5164, -52.6901) -> (-30.686, -52.6474)
  line L1194 (-27.2971, -52.6474) -> (-27.4667, -52.6901)
  line L1195 (-27.4667, -52.6901) -> (-27.5935, -52.817)
  line L1196 (-27.5935, -52.817) -> (-27.6363, -52.9865)
  line L1197 (-27.6363, -52.9865) -> (-27.5935, -53.1561)
  line L1198 (-27.5935, -53.1561) -> (-27.4667, -53.283)
  line L1199 (-27.4667, -53.283) -> (-27.2971, -53.3257)
  line L1200 (-18.6992, -41.9318) -> (-18.6992, -41.3389)
  line L1201 (-18.6992, -41.3389) -> (-18.6992, -40.6192)
  line L1202 (-18.6992, -40.6192) -> (-18.6992, -40.0263)
  line L1203 (-18.6992, -40.0263) -> (-15.2689, -40.0263)
  line L1204 (-15.2689, -40.0263) -> (-15.2689, -40.6192)
  line L1205 (-15.2689, -40.6192) -> (-15.2689, -41.3389)
  line L1206 (-15.2689, -41.3389) -> (-15.2689, -41.9318)
  line L1207 (-15.2689, -41.9318) -> (-18.6992, -41.9318)
  line L1208 (-17.3012, -40.2373) -> (-17.3012, -41.6781)
  line L1209 (-18.6992, -41.3389) -> (-18.5296, -41.2962)
  line L1210 (-18.5296, -41.2962) -> (-18.4028, -41.1693)
  line L1211 (-18.4028, -41.1693) -> (-18.3601, -40.9997)
  line L1212 (-18.3601, -40.9997) -> (-18.4028, -40.8301)
  line L1213 (-18.4028, -40.8301) -> (-18.5296, -40.7033)
  line L1214 (-18.5296, -40.7033) -> (-18.6992, -40.6192)
  line L1215 (-15.2689, -40.6192) -> (-15.4812, -40.7033)
  line L1216 (-15.4812, -40.7033) -> (-15.6081, -40.8301)
  line L1217 (-15.6081, -40.8301) -> (-15.6494, -40.9997)
  line L1218 (-15.6494, -40.9997) -> (-15.6081, -41.1693)
  line L1219 (-15.6081, -41.1693) -> (-15.4812, -41.2962)
  line L1220 (-15.4812, -41.2962) -> (-15.2689, -41.3389)
  line L1221 (16.7938, 33.1216) -> (20.3937, 33.1216)
  line L1222 (20.3937, 33.1216) -> (20.3937, 36.8911)
  line L1223 (20.3937, 36.8911) -> (16.7938, 36.8911)
  line L1224 (16.7938, 36.8911) -> (16.7938, 33.1216)
  line L1225 (-12.1764, -35.8749) -> (-8.5765, -35.8749)
  line L1226 (-8.5765, -35.8749) -> (-8.5765, -32.1054)
  line L1227 (-8.5765, -32.1054) -> (-12.1764, -32.1054)
  line L1228 (-12.1764, -32.1054) -> (-12.1764, -35.8749)
  line L1229 (8.1118, 13.9763) -> (7.4762, 13.3421)
  line L1230 (7.4762, 13.3421) -> (7.4762, 12.0709)
  line L1231 (7.4762, 12.0709) -> (8.1118, 11.4353)
  line L1232 (8.1118, 11.4353) -> (7.4762, 10.7997)
  line L1233 (7.4762, 10.7997) -> (7.4762, 9.5299)
  line L1234 (7.4762, 9.5299) -> (8.1118, 8.8943)
  line L1235 (8.1118, 8.8943) -> (7.4762, 8.2587)
  line L1236 (7.4762, 8.2587) -> (7.4762, 6.9889)
  line L1237 (7.4762, 6.9889) -> (8.1118, 6.3533)
  line L1238 (8.1118, 6.3533) -> (7.4762, 5.7177)
  line L1239 (7.4762, 5.7177) -> (7.4762, 4.4465)
  line L1240 (7.4762, 4.4465) -> (8.1118, 3.8122)
  line L1241 (8.1118, 3.8122) -> (7.4762, 3.1766)
  line L1242 (7.4762, 3.1766) -> (7.4762, 1.9054)
  line L1243 (7.4762, 1.9054) -> (8.1118, 1.2698)
  line L1244 (8.1118, 1.2698) -> (7.4762, 0.6356)
  line L1245 (7.4762, 0.6356) -> (7.4762, -0.6356)
  line L1246 (7.4762, -0.6356) -> (8.1118, -1.2712)
  line L1247 (8.1118, 13.9763) -> (11.9227, 13.9763)
  line L1248 (11.9227, 13.9763) -> (12.5583, 13.3421)
  line L1249 (12.5583, 13.3421) -> (12.5583, 12.0709)
  line L1250 (12.5583, 12.0709) -> (11.9227, 11.4353)
  line L1251 (11.9227, 11.4353) -> (12.5583, 10.7997)
  line L1252 (12.5583, 10.7997) -> (12.5583, 9.5299)
  line L1253 (12.5583, 9.5299) -> (11.9227, 8.8943)
  line L1254 (11.9227, 8.8943) -> (12.5583, 8.2587)
  line L1255 (12.5583, 8.2587) -> (12.5583, 6.9889)
  line L1256 (12.5583, 6.9889) -> (11.9227, 6.3533)
  line L1257 (11.9227, 6.3533) -> (12.5583, 5.7177)
  line L1258 (12.5583, 5.7177) -> (12.5583, 4.4465)
  line L1259 (12.5583, 4.4465) -> (11.9227, 3.8122)
  line L1260 (11.9227, 3.8122) -> (12.5583, 3.1766)
  line L1261 (12.5583, 3.1766) -> (12.5583, 1.9054)
  line L1262 (12.5583, 1.9054) -> (11.9227, 1.2698)
  line L1263 (11.9227, 1.2698) -> (12.5583, 0.6356)
  line L1264 (12.5583, 0.6356) -> (12.5583, -0.6356)
  line L1265 (12.5583, -0.6356) -> (11.9227, -1.2712)
  line L1266 (11.9227, -1.2712) -> (12.5583, -1.9068)
  line L1267 (12.5583, -1.9068) -> (12.5583, -3.1766)
  line L1268 (12.5583, -3.1766) -> (11.9227, -3.8122)
  line L1269 (11.9227, -3.8122) -> (12.5583, -4.4478)
  line L1270 (12.5583, -4.4478) -> (12.5583, -5.7177)
  line L1271 (12.5583, -5.7177) -> (11.9227, -6.3533)
  line L1272 (11.9227, -6.3533) -> (12.5583, -6.9889)
  line L1273 (12.5583, -6.9889) -> (12.5583, -8.2601)
  line L1274 (12.5583, -8.2601) -> (11.9227, -8.8943)
  line L1275 (11.9227, -8.8943) -> (12.5583, -9.5299)
  line L1276 (12.5583, -9.5299) -> (12.5583, -10.8011)
  line L1277 (12.5583, -10.8011) -> (11.9227, -11.4367)
  line L1278 (8.1118, -11.4367) -> (7.4762, -10.8011)
  line L1279 (7.4762, -10.8011) -> (7.4762, -9.5299)
  line L1280 (8.1118, -8.8943) -> (7.4762, -9.5299)
  line L1281 (8.1118, -8.8943) -> (7.4762, -8.2601)
  line L1282 (7.4762, -8.2601) -> (7.4762, -6.9889)
  line L1283 (8.1118, -6.3533) -> (7.4762, -6.9889)
  line L1284 (8.1118, -6.3533) -> (7.4762, -5.7177)
  line L1285 (7.4762, -5.7177) -> (7.4762, -4.4478)
  line L1286 (8.1118, -3.8122) -> (7.4762, -4.4478)
  line L1287 (8.1118, -3.8122) -> (7.4762, -3.1766)
  line L1288 (7.4762, -3.1766) -> (7.4762, -1.9068)
  line L1289 (8.1118, -1.2712) -> (7.4762, -1.9068)
  line L1290 (11.9227, 11.4353) -> (8.1118, 11.4353)
  line L1291 (11.9227, 8.8943) -> (8.1118, 8.8943)
  line L1292 (11.9227, 6.3533) -> (8.1118, 6.3533)
  line L1293 (11.9227, 3.8122) -> (8.1118, 3.8122)
  line L1294 (11.9227, 1.2698) -> (8.1118, 1.2698)
  line L1295 (11.9227, -1.2712) -> (8.1118, -1.2712)
  line L1296 (11.9227, -3.8122) -> (8.1118, -3.8122)
  line L1297 (11.9227, -6.3533) -> (8.1118, -6.3533)
  line L1298 (11.9227, -8.8943) -> (8.1118, -8.8943)
  line L1299 (11.9227, -11.4367) -> (8.1118, -11.4367)
  line L1300 (11.9227, -11.4367) -> (12.5583, -12.0709)
  line L1301 (12.5583, -12.0709) -> (12.5583, -13.3421)
  line L1302 (12.5583, -13.3421) -> (11.9227, -13.9777)
  line L1303 (8.1118, -13.9777) -> (7.4762, -13.3421)
  line L1304 (7.4762, -13.3421) -> (7.4762, -12.0709)
  line L1305 (8.1118, -11.4367) -> (7.4762, -12.0709)
  line L1306 (11.9227, -13.9777) -> (8.1118, -13.9777)
  line L1307 (28.2305, 16.0941) -> (28.2305, 15.1207)
  line L1308 (26.0273, 15.1207) -> (26.0273, 16.0941)
  line L1309 (34.2018, 14.5278) -> (34.2018, 13.5103)
  line L1310 (32, 13.5103) -> (32, 14.5278)
  line L1311 (41.6981, 15.1207) -> (41.6981, 16.0941)
  spline S100 degree 3 poles (-12.8975, -6.4387) (-12.8975, -7.0316) (-13.4048, -7.539) (-13.9977, -7.539) knots 0 0 0 0 1 1 1 1
  line L1312 (-12.8975, -6.4387) -> (-12.8975, -7.0316) construction
  line L1313 (-12.8975, -7.0316) -> (-13.4048, -7.539) construction
  line L1314 (-13.4048, -7.539) -> (-13.9977, -7.539) construction
  spline S101 degree 3 poles (-13.9977, -7.539) (-14.5906, -7.539) (-15.0993, -7.0316) (-15.0993, -6.4387) knots 0 0 0 0 1 1 1 1
  line L1315 (-13.9977, -7.539) -> (-14.5906, -7.539) construction
  line L1316 (-14.5906, -7.539) -> (-15.0993, -7.0316) construction
  line L1317 (-15.0993, -7.0316) -> (-15.0993, -6.4387) construction
  spline S102 degree 3 poles (-15.0993, -6.4387) (-15.0993, -5.8459) (-14.5906, -5.3371) (-13.9977, -5.3371) knots 0 0 0 0 1 1 1 1
  line L1318 (-15.0993, -6.4387) -> (-15.0993, -5.8459) construction
  line L1319 (-15.0993, -5.8459) -> (-14.5906, -5.3371) construction
  line L1320 (-14.5906, -5.3371) -> (-13.9977, -5.3371) construction
  spline S103 degree 3 poles (-13.9977, -5.3371) (-13.4048, -5.3371) (-12.8975, -5.8459) (-12.8975, -6.4387) knots 0 0 0 0 1 1 1 1
  line L1321 (-13.9977, -5.3371) -> (-13.4048, -5.3371) construction
  line L1322 (-13.4048, -5.3371) -> (-12.8975, -5.8459) construction
  line L1323 (-12.8975, -5.8459) -> (-12.8975, -6.4387) construction
  line L1324 (43.9013, 16.0941) -> (43.9013, 15.1207)
  spline S104 degree 3 poles (-12.8975, 6.3533) (-12.8975, 5.7604) (-13.4048, 5.2516) (-13.9977, 5.2516) knots 0 0 0 0 1 1 1 1
  line L1325 (-12.8975, 6.3533) -> (-12.8975, 5.7604) construction
  line L1326 (-12.8975, 5.7604) -> (-13.4048, 5.2516) construction
  line L1327 (-13.4048, 5.2516) -> (-13.9977, 5.2516) construction
  spline S105 degree 3 poles (-13.9977, 5.2516) (-14.5906, 5.2516) (-15.0993, 5.7604) (-15.0993, 6.3533) knots 0 0 0 0 1 1 1 1
  line L1328 (-13.9977, 5.2516) -> (-14.5906, 5.2516) construction
  line L1329 (-14.5906, 5.2516) -> (-15.0993, 5.7604) construction
  line L1330 (-15.0993, 5.7604) -> (-15.0993, 6.3533) construction
  spline S106 degree 3 poles (-15.0993, 6.3533) (-15.0993, 6.9461) (-14.5906, 7.4535) (-13.9977, 7.4535) knots 0 0 0 0 1 1 1 1
  line L1331 (-15.0993, 6.3533) -> (-15.0993, 6.9461) construction
  line L1332 (-15.0993, 6.9461) -> (-14.5906, 7.4535) construction
  line L1333 (-14.5906, 7.4535) -> (-13.9977, 7.4535) construction
  spline S107 degree 3 poles (-13.9977, 7.4535) (-13.4048, 7.4535) (-12.8975, 6.9461) (-12.8975, 6.3533) knots 0 0 0 0 1 1 1 1
  line L1334 (-13.9977, 7.4535) -> (-13.4048, 7.4535) construction
  line L1335 (-13.4048, 7.4535) -> (-12.8975, 6.9461) construction
  line L1336 (-12.8975, 6.9461) -> (-12.8975, 6.3533) construction
  spline S108 degree 3 poles (5.0193, 31.0038) (5.0193, 30.7074) (4.807, 30.4951) (4.5106, 30.4951) knots 0 0 0 0 1 1 1 1
  line L1337 (5.0193, 31.0038) -> (5.0193, 30.7074) construction
  line L1338 (5.0193, 30.7074) -> (4.807, 30.4951) construction
  line L1339 (4.807, 30.4951) -> (4.5106, 30.4951) construction
  spline S109 degree 3 poles (4.5106, 30.4951) (4.2141, 30.4951) (4.0032, 30.7074) (4.0032, 31.0038) knots 0 0 0 0 1 1 1 1
  line L1340 (4.5106, 30.4951) -> (4.2141, 30.4951) construction
  line L1341 (4.2141, 30.4951) -> (4.0032, 30.7074) construction
  line L1342 (4.0032, 30.7074) -> (4.0032, 31.0038) construction
  spline S110 degree 3 poles (4.0032, 31.0038) (4.0032, 31.3003) (4.2141, 31.5112) (4.5106, 31.5112) knots 0 0 0 0 1 1 1 1
  line L1343 (4.0032, 31.0038) -> (4.0032, 31.3003) construction
  line L1344 (4.0032, 31.3003) -> (4.2141, 31.5112) construction
  line L1345 (4.2141, 31.5112) -> (4.5106, 31.5112) construction
  spline S111 degree 3 poles (4.5106, 31.5112) (4.807, 31.5112) (5.0193, 31.3003) (5.0193, 31.0038) knots 0 0 0 0 1 1 1 1
  line L1346 (4.5106, 31.5112) -> (4.807, 31.5112) construction
  line L1347 (4.807, 31.5112) -> (5.0193, 31.3003) construction
  line L1348 (5.0193, 31.3003) -> (5.0193, 31.0038) construction
  spline S112 degree 3 poles (-3.9604, 31.0038) (-3.9604, 30.7074) (-4.1714, 30.4951) (-4.4678, 30.4951) knots 0 0 0 0 1 1 1 1
  line L1349 (-3.9604, 31.0038) -> (-3.9604, 30.7074) construction
  line L1350 (-3.9604, 30.7074) -> (-4.1714, 30.4951) construction
  line L1351 (-4.1714, 30.4951) -> (-4.4678, 30.4951) construction
  spline S113 degree 3 poles (-4.4678, 30.4951) (-4.7643, 30.4951) (-4.9766, 30.7074) (-4.9766, 31.0038) knots 0 0 0 0 1 1 1 1
  line L1352 (-4.4678, 30.4951) -> (-4.7643, 30.4951) construction
  line L1353 (-4.7643, 30.4951) -> (-4.9766, 30.7074) construction
  line L1354 (-4.9766, 30.7074) -> (-4.9766, 31.0038) construction
  spline S114 degree 3 poles (-4.9766, 31.0038) (-4.9766, 31.3003) (-4.7643, 31.5112) (-4.4678, 31.5112) knots 0 0 0 0 1 1 1 1
  line L1355 (-4.9766, 31.0038) -> (-4.9766, 31.3003) construction
  line L1356 (-4.9766, 31.3003) -> (-4.7643, 31.5112) construction
  line L1357 (-4.7643, 31.5112) -> (-4.4678, 31.5112) construction
  spline S115 degree 3 poles (-4.4678, 31.5112) (-4.1714, 31.5112) (-3.9604, 31.3003) (-3.9604, 31.0038) knots 0 0 0 0 1 1 1 1
  line L1358 (-4.4678, 31.5112) -> (-4.1714, 31.5112) construction
  line L1359 (-4.1714, 31.5112) -> (-3.9604, 31.3003) construction
  line L1360 (-3.9604, 31.3003) -> (-3.9604, 31.0038) construction
  spline S116 degree 3 poles (-3.9604, -31.0038) (-3.9604, -31.3003) (-4.1714, -31.5126) (-4.4678, -31.5126) knots 0 0 0 0 1 1 1 1
  line L1361 (-3.9604, -31.0038) -> (-3.9604, -31.3003) construction
  line L1362 (-3.9604, -31.3003) -> (-4.1714, -31.5126) construction
  line L1363 (-4.1714, -31.5126) -> (-4.4678, -31.5126) construction
  spline S117 degree 3 poles (-4.4678, -31.5126) (-4.7643, -31.5126) (-4.9766, -31.3003) (-4.9766, -31.0038) knots 0 0 0 0 1 1 1 1
  line L1364 (-4.4678, -31.5126) -> (-4.7643, -31.5126) construction
  line L1365 (-4.7643, -31.5126) -> (-4.9766, -31.3003) construction
  line L1366 (-4.9766, -31.3003) -> (-4.9766, -31.0038) construction
  spline S118 degree 3 poles (-4.9766, -31.0038) (-4.9766, -30.7074) (-4.7643, -30.4965) (-4.4678, -30.4965) knots 0 0 0 0 1 1 1 1
  line L1367 (-4.9766, -31.0038) -> (-4.9766, -30.7074) construction
  line L1368 (-4.9766, -30.7074) -> (-4.7643, -30.4965) construction
  line L1369 (-4.7643, -30.4965) -> (-4.4678, -30.4965) construction
  spline S119 degree 3 poles (-4.4678, -30.4965) (-4.1714, -30.4965) (-3.9604, -30.7074) (-3.9604, -31.0038) knots 0 0 0 0 1 1 1 1
  line L1370 (-4.4678, -30.4965) -> (-4.1714, -30.4965) construction
  line L1371 (-4.1714, -30.4965) -> (-3.9604, -30.7074) construction
  line L1372 (-3.9604, -30.7074) -> (-3.9604, -31.0038) construction
  spline S120 degree 3 poles (5.0193, -31.0038) (5.0193, -31.3003) (4.807, -31.5126) (4.5106, -31.5126) knots 0 0 0 0 1 1 1 1
  line L1373 (5.0193, -31.0038) -> (5.0193, -31.3003) construction
  line L1374 (5.0193, -31.3003) -> (4.807, -31.5126) construction
  line L1375 (4.807, -31.5126) -> (4.5106, -31.5126) construction
  spline S121 degree 3 poles (4.5106, -31.5126) (4.2141, -31.5126) (4.0032, -31.3003) (4.0032, -31.0038) knots 0 0 0 0 1 1 1 1
  line L1376 (4.5106, -31.5126) -> (4.2141, -31.5126) construction
  line L1377 (4.2141, -31.5126) -> (4.0032, -31.3003) construction
  line L1378 (4.0032, -31.3003) -> (4.0032, -31.0038) construction
  spline S122 degree 3 poles (4.0032, -31.0038) (4.0032, -30.7074) (4.2141, -30.4965) (4.5106, -30.4965) knots 0 0 0 0 1 1 1 1
  line L1379 (4.0032, -31.0038) -> (4.0032, -30.7074) construction
  line L1380 (4.0032, -30.7074) -> (4.2141, -30.4965) construction
  line L1381 (4.2141, -30.4965) -> (4.5106, -30.4965) construction
  spline S123 degree 3 poles (4.5106, -30.4965) (4.807, -30.4965) (5.0193, -30.7074) (5.0193, -31.0038) knots 0 0 0 0 1 1 1 1
  line L1382 (4.5106, -30.4965) -> (4.807, -30.4965) construction
  line L1383 (4.807, -30.4965) -> (5.0193, -30.7074) construction
  line L1384 (5.0193, -30.7074) -> (5.0193, -31.0038) construction
  spline S124 degree 3 poles (-7.7299, -44.0068) (-7.7299, -44.7279) (-8.2801, -45.278) (-8.9998, -45.278) knots 0 0 0 0 1 1 1 1
  line L1385 (-7.7299, -44.0068) -> (-7.7299, -44.7279) construction
  line L1386 (-7.7299, -44.7279) -> (-8.2801, -45.278) construction
  line L1387 (-8.2801, -45.278) -> (-8.9998, -45.278) construction
  spline S125 degree 3 poles (-8.9998, -45.278) (-9.7208, -45.278) (-10.271, -44.7279) (-10.271, -44.0068) knots 0 0 0 0 1 1 1 1
  line L1388 (-8.9998, -45.278) -> (-9.7208, -45.278) construction
  line L1389 (-9.7208, -45.278) -> (-10.271, -44.7279) construction
  line L1390 (-10.271, -44.7279) -> (-10.271, -44.0068) construction
  spline S126 degree 3 poles (-10.271, -44.0068) (-10.271, -43.2871) (-9.7208, -42.737) (-8.9998, -42.737) knots 0 0 0 0 1 1 1 1
  line L1391 (-10.271, -44.0068) -> (-10.271, -43.2871) construction
  line L1392 (-10.271, -43.2871) -> (-9.7208, -42.737) construction
  line L1393 (-9.7208, -42.737) -> (-8.9998, -42.737) construction
  spline S127 degree 3 poles (-8.9998, -42.737) (-8.2801, -42.737) (-7.7299, -43.2871) (-7.7299, -44.0068) knots 0 0 0 0 1 1 1 1
  line L1394 (-8.9998, -42.737) -> (-8.2801, -42.737) construction
  line L1395 (-8.2801, -42.737) -> (-7.7299, -43.2871) construction
  line L1396 (-7.7299, -43.2871) -> (-7.7299, -44.0068) construction
  spline S128 degree 3 poles (10.271, -44.0068) (10.271, -44.7279) (9.7208, -45.278) (9.0011, -45.278) knots 0 0 0 0 1 1 1 1
  line L1397 (10.271, -44.0068) -> (10.271, -44.7279) construction
  line L1398 (10.271, -44.7279) -> (9.7208, -45.278) construction
  line L1399 (9.7208, -45.278) -> (9.0011, -45.278) construction
  spline S129 degree 3 poles (9.0011, -45.278) (8.28, -45.278) (7.7299, -44.7279) (7.7299, -44.0068) knots 0 0 0 0 1 1 1 1
  line L1400 (9.0011, -45.278) -> (8.28, -45.278) construction
  line L1401 (8.28, -45.278) -> (7.7299, -44.7279) construction
  line L1402 (7.7299, -44.7279) -> (7.7299, -44.0068) construction
  spline S130 degree 3 poles (7.7299, -44.0068) (7.7299, -43.2871) (8.28, -42.737) (9.0011, -42.737) knots 0 0 0 0 1 1 1 1
  line L1403 (7.7299, -44.0068) -> (7.7299, -43.2871) construction
  line L1404 (7.7299, -43.2871) -> (8.28, -42.737) construction
  line L1405 (8.28, -42.737) -> (9.0011, -42.737) construction
  spline S131 degree 3 poles (9.0011, -42.737) (9.7208, -42.737) (10.271, -43.2871) (10.271, -44.0068) knots 0 0 0 0 1 1 1 1
  line L1406 (9.0011, -42.737) -> (9.7208, -42.737) construction
  line L1407 (9.7208, -42.737) -> (10.271, -43.2871) construction
  line L1408 (10.271, -43.2871) -> (10.271, -44.0068) construction
  spline S132 degree 3 poles (-50.3814, -49.9795) (-50.3814, -50.8688) (-51.1011, -51.5885) (-51.9904, -51.5885) knots 0 0 0 0 1 1 1 1
  line L1409 (-50.3814, -49.9795) -> (-50.3814, -50.8688) construction
  line L1410 (-50.3814, -50.8688) -> (-51.1011, -51.5885) construction
  line L1411 (-51.1011, -51.5885) -> (-51.9904, -51.5885) construction
  spline S133 degree 3 poles (-51.9904, -51.5885) (-52.8797, -51.5885) (-53.6008, -50.8688) (-53.6008, -49.9795) knots 0 0 0 0 1 1 1 1
  line L1412 (-51.9904, -51.5885) -> (-52.8797, -51.5885) construction
  line L1413 (-52.8797, -51.5885) -> (-53.6008, -50.8688) construction
  line L1414 (-53.6008, -50.8688) -> (-53.6008, -49.9795) construction
  spline S134 degree 3 poles (-53.6008, -49.9795) (-53.6008, -49.0902) (-52.8797, -48.3705) (-51.9904, -48.3705) knots 0 0 0 0 1 1 1 1
  line L1415 (-53.6008, -49.9795) -> (-53.6008, -49.0902) construction
  line L1416 (-53.6008, -49.0902) -> (-52.8797, -48.3705) construction
  line L1417 (-52.8797, -48.3705) -> (-51.9904, -48.3705) construction
  spline S135 degree 3 poles (-51.9904, -48.3705) (-51.1011, -48.3705) (-50.3814, -49.0902) (-50.3814, -49.9795) knots 0 0 0 0 1 1 1 1
  line L1418 (-51.9904, -48.3705) -> (-51.1011, -48.3705) construction